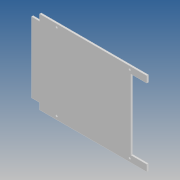
# Autodesk Inventor part: KB33-046-004-018 - Полка электроники
Saved by Autodesk Inventor 2020 (Build 240168000, 168)
## iProperties
Created: 2021-06-26
Part Number: KB33-046-004-018 - Полка электроники
Material: Типовые
Document SubType Name: Modeling
Designer: Петров Иван
Mass: 183.976 g
Surface Area: 962.119 cm^2
Volume: 183.976 cm^3
Density: 1 g/cm^3
Appearance: По умолчанию
Author: Петров Иван
Autodesk Inventor part; units mm, degrees
ref_plane "YZ Plane" through (0, 0, 0) normal (1, 0, 0) x (0, 1, 0)
ref_plane "XZ Plane" through (0, 0, 0) normal (0, 1, 0) x (-1, 0, 0)
ref_plane "XY Plane" through (0, 0, 0) normal (0, 0, 1) x (1, 0, 0)
sketch "Эскиз1" plane through (0, 0, 0) normal (0, 0, 1) x (1, 0, 0)
  circle A0 centre (196.5682, -22.5) radius 2 projected
  circle A1 centre (25, -22.5) radius 2 projected
  circle A2 centre (25, 157.5) radius 2 projected
  circle A3 centre (196.5682, 157.5) radius 2 projected
  line L0 (236.5682, -15) -> (236.5682, -30) projected
  line L1 (236.5682, 150) -> (236.5682, 165) projected
  line L2 (-15, -15) -> (-15, -30) projected
  line L3 (-34.0192, -15) -> (-15, -15) projected
  line L4 (-15, 150) -> (-15, 165) projected
  line L5 (-34.0192, 150) -> (-15, 150) projected
  line L6 (-34.0192, 150) -> (-15, 150)
  line L7 (-15, 150) -> (-15, -15)
  line L8 (-15, -15) -> (-34.0192, -15)
  line L9 (-34.0192, -15) -> (-34.0192, 150)
  line L10 (236.5682, 165) -> (-15, 165)
  line L11 (-15, 165) -> (-15, -30)
  line L12 (-15, -30) -> (236.5682, -30)
  line L13 (236.5682, -30) -> (236.5682, 165)
  point P0 (0, 0)
  constraints: 16 end point, 4 parallel, 2 horizontal, 2 perpendicular
extrude "Выдавливание1" add sketch "Эскиз1" along normal blind 4
sketch "Эскиз2" plane through (0, 0, 4) normal (0, 0, 1) x (1, 0, 0)
  line L0 (236.5682, -30) -> (236.5682, 165) projected
  line L1 (236.5682, 150) -> (199.2972, 150)
  line L2 (199.2972, 150) -> (199.2972, -15)
  line L3 (199.2972, -15) -> (236.5682, -15)
  line L4 (236.5682, -15) -> (236.5682, 150)
  line L5 (-15, 150) -> (-34.0192, 150) projected
  point P0 (0, 0)
  point P1 (-24.5096, 150)
  point P2 (-15, -15)
  constraints: 8 end point, 2 horizontal alignment, 2 parallel, 1 horizontal, 1 midpoint, 1 perpendicular, 1 point on line
extrude "Выдавливание2" cut sketch "Эскиз2" against normal blind 4
